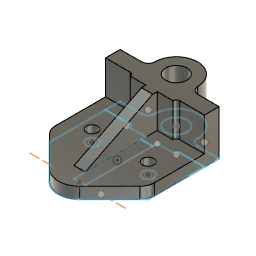
Piece-3 v4 (Autodesk Fusion 360 design; units mm, degrees)
Autodesk Fusion 360 part; units mm, degrees
sketch "Main" plane through (0, 0, 0) normal (0, 0, 1) x (1, 0, 0)
  line L0 (-44, 33.5) -> (-44, -16.3701)
  line L1 (44, -16.3701) -> (44, 33.5)
  line L2 (-25, 33.5) -> (-25, -33.5) construction
  line L3 (25, 33.5) -> (25, -33.5) construction
  line L4 (-44, 2.5) -> (44, 2.5) construction
  circle A0 centre (-25, 2.5) radius 5
  arc A1 (-13.435, -46.935) -> (13.435, -46.935) centre (0, -33.5) ccw
  line L5 (-26.8701, -33.5) -> (-25, -33.5)
  circle A2 centre (25, 2.5) radius 5
  line L6 (0, -33.5) -> (-13.435, -46.935) construction
  line L7 (0, -33.5) -> (19, -33.5) construction
  line L8 (0, -33.5) -> (13.435, -46.935) construction
  line L9 (-13.435, -46.935) -> (-44, -16.3701)
  line L10 (13.435, -46.935) -> (44, -16.3701)
  line L11 (-44, -33.5) -> (-26.8701, -33.5) construction
  line L12 (-25, -33.5) -> (44, -33.5) construction
  line L13 (44, 33.5) -> (44, 46.5)
  line L14 (-44, 46.5) -> (-44, 33.5)
  arc A3 (-19, 30.5) -> (-22, 33.5) centre (-22, 30.5) ccw
  arc A4 (22, 33.5) -> (19, 30.5) centre (22, 30.5) ccw
  line L15 (-44, 33.5) -> (-22, 33.5)
  line L16 (22, 33.5) -> (44, 33.5)
  line L17 (44, 33.5) -> (22, 33.5)
  line L18 (-22, 33.5) -> (-44, 33.5)
  line L19 (-5, 30.5) -> (-5, -33.5) construction
  line L20 (5, 30.5) -> (5, -33.5) construction
  line L21 (5, 30.5) -> (5, 26.5)
  line L22 (5, 26.5) -> (-5, 26.5)
  line L23 (-5, 26.5) -> (-5, 30.5)
  line L24 (19, 30.5) -> (5, 30.5)
  line L25 (-5, 30.5) -> (-19, 30.5)
  line L26 (-5, 26.5) -> (5, 26.5)
  line L27 (5, 26.5) -> (5, -33.5)
  line L28 (5, -33.5) -> (-5, -33.5)
  line L29 (-5, -33.5) -> (-5, 26.5)
  line L30 (33, 33.5) -> (33, 52.5) construction
  line L31 (33, 52.5) -> (0, 52.5) construction
  circle A5 centre (0, 52.5) radius 9.5
  line L32 (44, 46.5) -> (25, 46.5)
  arc A6 (19, 52.5) -> (25, 46.5) centre (25, 52.5) ccw
  arc A7 (-25, 46.5) -> (-19, 52.5) centre (-25, 52.5) ccw
  arc A8 (19, 52.5) -> (-19, 52.5) centre (0, 52.5) ccw
  line L33 (-25, 46.5) -> (-44, 46.5)
  dimension "d3" = 50
  dimension "d4" = 19
  dimension "d5" = 31
  dimension "d6" = 36
  dimension "d7" = 10
  dimension "d8" = 19
  dimension "d9" = 10
  dimension "d10" = 135
  dimension "d14" = 88
  dimension "d15" = 13
  dimension "d19" = 3
  dimension "d20" = 3
  dimension "d21" = 10
  dimension "d22" = 20
  dimension "d23" = 4
  dimension "d24" = 19
  dimension "d25" = 19
  dimension "d26" = 19
  dimension "d27" = 6
  dimension "d28" = 6
  constraint horizontal L17
  constraint perpendicular L0 L17
  constraint parallel L5 L17
  constraint parallel L0 L1
  constraint coincident L2.start L17
  constraint perpendicular L2 L5
  constraint coincident L3.start L17
  constraint coincident L3.end L5
  constraint perpendicular L3 L5
  constraint coincident L0 L4.start
  constraint coincident L1 L4.end
  constraint perpendicular L1 L4
  constraint coincident L0 L11.start
  constraint coincident L1 L12.end
  constraint perpendicular L1 L11
  constraint coincident L4 A0.centre
  constraint coincident L2 A0.centre
  constraint coincident L3 A2.centre
  constraint coincident L4 A2.centre
  constraint horizontal L7
  constraint coincident A1.centre L6.start
  constraint perpendicular L6 L8
  constraint perpendicular L6 L9
  constraint tangent A1 L10
  constraint coincident L9 L5.start
  constraint collinear L11 L12
  constraint coincident A1.centre L11
  constraint horizontal L15
  constraint vertical L13
  constraint horizontal L32
  constraint vertical L14
  constraint horizontal L24
  constraint tangent A3 L17
  constraint coincident A3.end L17
  constraint tangent A4 L17
  constraint collinear L15 L16
  constraint collinear L17 L18
  constraint coincident L19.start L24
  constraint coincident L12 L19.end
  constraint perpendicular L12 L19
  constraint coincident L12 L20.end
  constraint perpendicular L12 L20
  constraint vertical L21
  constraint horizontal L22
  constraint vertical L23
  constraint coincident L20 L21.end
  constraint collinear L24 L25
  constraint horizontal L26
  constraint vertical L27
  constraint horizontal L28
  constraint vertical L29
  constraint midpoint L17 L30.start
  constraint perpendicular L17 L30
  constraint perpendicular L30 L31
  constraint coincident L31.end A5.centre
  constraint concentric A5 A8
  constraint tangent A6 A8
  constraint tangent L32 A6
  constraint tangent A7 A8
  constraint coincident L31 A6.start
  measures "d3" distance of L2 L3
  measures "d4" distance of L0 L2
  measures "d5" distance of L4 L17
  measures "d6" distance of L4 L11 L1.end
  measures "d7" diameter of A0
  measures "d8" radius of A1
  measures "d9" diameter of A2
  measures "d10" angle of L6 L7
  measures "d14" distance of L0.start L1.end
  measures "d15" distance of L0.start L14.start
  measures "d19" radius of A3
  measures "d20" radius of A4
  measures "d21" distance of L19 L20
  measures "d22" distance of L2 L19
  measures "d23" distance of L19.start L22.end
  measures "d24" distance of L30.start L30.end
  measures "d25" diameter of A5
  measures "d26" radius of A8
  measures "d27" radius of A6
  measures "d28" radius of A7
extrude "Extrude1" add sketch "Main" along normal blind 10 contours L0 L1 A1 L9 L10 A3 A4 L15 L16 L17 L18 L21 L23 L24 L25 L27 L28 L29 makes body 1
fillet "Fillet1" radius 13 2 edges at (44, -16.3701, 5) (-44, -16.3701, 5) on bodies 1
extrude "Extrude2" add sketch "Main" along normal blind 40 separate body contours L13 L14 A3 A4 L15 L16 L17 L18 L21 L22 L23 L24 L25 L26 L32 A6 A7 A8 L33 makes body 2
extrude "Extrude3" add sketch "Main" along normal blind 40 separate body contours L22 L26 L27 L28 L29 makes body 3
draft "Draft1" angle 26.5 neutral plane through (5, 26.5, 0) pull (0, -1, 0) 1 faces at (-1.6667, 6.5, 40) on bodies 3
combine "Combine1" operation add target body 2 tool bodies 1 3
equation "d4 = ( ( 88 - 50 ) / 2 ) * 1 mm"
equation "d10 = 90 deg + 45 deg"
equation "d23 = 20 mm - 13 mm - 3 mm"
named bodies: "Lower", "Piece-3", "Slope"
